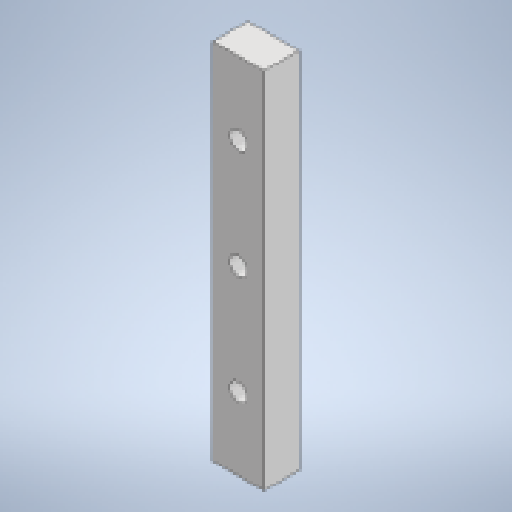
# Autodesk Inventor part: MGN7c_50mm_rail
Saved by Autodesk Inventor 2024.1 (Build 281209000, 209)
## iProperties
Created: 2023-09-16
Part Number: MGN7c_50mm_rail
Material: Generic
Document SubType Name: Modeling
Designer: l1534
Density: 1 g/cm^3
Appearance: Default
Author: l1534
Autodesk Inventor part; units mm, degrees
ref_plane "YZ Plane" through (0, 0, 0) normal (1, 0, 0) x (0, 1, 0)
ref_plane "XZ Plane" through (0, 0, 0) normal (0, 1, 0) x (-1, 0, 0)
ref_plane "XY Plane" through (0, 0, 0) normal (0, 0, 1) x (1, 0, 0)
sketch "Sketch1" plane through (0, 0, 0) normal (0, 1, 0) x (-1, 0, 0)
  line L0 (3.8413, -2.6197) -> (-3.1587, -2.6197)
  line L1 (-3.1587, -2.6197) -> (-3.1587, 2.1803)
  line L2 (-3.1587, 2.1803) -> (3.8413, 2.1803)
  line L3 (3.8413, 2.1803) -> (3.8413, -2.6197)
  point P0 (0, 0)
  dimension "d0" = 4.8
  dimension "d1" = 7
  constraints: 8 end point, 2 parallel, 1 horizontal, 1 perpendicular
  measures "d0" distance of L0.end L1.end
  measures "d1" distance of L0.start L0.end
extrude "Extrusion1" add sketch "Sketch1" along normal blind 50
sketch "Sketch2" plane through (3.1587, 0, -2.6197) normal (0, 0, -1) x (-1, 0, 0)
  circle A0 centre (3.5, 10) radius 1.2
  line L0 (0, 0) -> (7, 0) projected
  line L1 (7, 0) -> (7, 50) projected
  circle A1 centre (3.5, 25) radius 1.2
  circle A2 centre (3.5, 40) radius 1.2
  point P0 (3.1587, 0)
  dimension "d4" = 2.4
  dimension "d5" = 10
  dimension "d6" = 3.5
  dimension "d9" = 15
  constraints: 3 centre point, 1 vertical, 4 other
  measures "d4" diameter of A0
  measures "d5" distance from line of L0 A0.centre
  measures "d6" distance from line of L1 A0.centre
  measures "d9" distance of A0.centre A1.centre
extrude "Extrusion2" cut sketch "Sketch2" against normal through all
sketch "Sketch3" plane through (3.1587, 0, -2.6197) normal (0, 0, -1) x (-1, 0, 0)
  circle A0 centre (3.5, 40) radius 1.2 projected
  circle A1 centre (3.5, 40) radius 2.1
  circle A2 centre (3.5, 25) radius 1.2 projected
  circle A3 centre (3.5, 25) radius 2.1
  circle A4 centre (3.5, 10) radius 1.2 projected
  circle A5 centre (3.5, 10) radius 2.1
  point P0 (3.1587, 0)
  dimension "d16" = 4.2
  dimension "d17" = 4.2
  dimension "d18" = 4.2
  constraints: 3 centre point, 3 coincident
  measures "d16" diameter of A1
  measures "d17" diameter of A3
  measures "d18" diameter of A5
extrude "Extrusion3" cut sketch "Sketch3" against normal blind 2.3 contours A0 | A1 | A2 | A3 | A4 | A5
body "Solid1"
